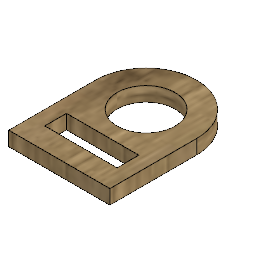
Exercise_1 (Autodesk Fusion 360 design; units mm, degrees)
Autodesk Fusion 360 part; units mm, degrees
sketch "Sketch1" plane through (0, 0, 0) normal (0, 0, 1) x (1, 0, 0)
  line L0 (0, 0) -> (70, 0)
  line L1 (70, 0) -> (70, 60)
  line L2 (0, 60) -> (0, 0)
  arc A0 (70, 60) -> (0, 60) centre (35, 60) ccw
  circle A1 centre (35, 60) radius 20
  line L3 (10, 30) -> (60, 30)
  line L4 (60, 30) -> (60, 15)
  line L5 (60, 15) -> (10, 15)
  line L6 (10, 15) -> (10, 30)
  dimension "d1" = 70
  dimension "d2" = 60
  dimension "d3" = 40
  dimension "d4" = 50
  dimension "d5" = 15
  dimension "d6" = 10
  dimension "d7" = 15
  constraint horizontal L0
  constraint vertical L1
  constraint vertical L2
  constraint coincident L0.start L2.end
  constraint concentric A0 A1
  constraint horizontal L3
  constraint vertical L4
  constraint horizontal L5
  constraint vertical L6
  measures "d1" distance of L0.start L0.end
  measures "d2" distance of L0.start L2.start
  measures "d3" diameter of A1
  measures "d4" distance of L3.start L3.end
  measures "d5" distance of L3 L5
  measures "d6" distance of L2 L6
  measures "d7" distance of L0 L5
extrude "Extrude1" add sketch "Sketch1" along normal blind 10
